Autodesk Inventor part; units mm, degrees
(part 3 of 3)
  line L1377 (0, -93.0469) -> (0, -126.0469) construction
  arc A64 (0, -126.0469) -> (6, -132.0469) centre (6, -126.0469) ccw construction
  line L1378 (16.4732, -132.0469) -> (6, -132.0469) construction
  circle A65 centre (10, -122.0469) radius 1.6 construction
  circle A66 centre (10, 47.9531) radius 1.6 construction
  circle A67 centre (27.5, -71.0469) radius 1.6 construction
  circle A68 centre (72.5, 11.9531) radius 1.6 construction
  circle A69 centre (27.5, 11.9531) radius 1.6 construction
  circle A70 centre (50, 69.0653) radius 1.6 construction
  arc A71 (58, 66.0653) -> (55, 66.0653) centre (56.5, 66.0653) ccw construction
  line L1379 (58, 66.0653) -> (58, 63.0653) construction
  arc A72 (55, 63.0653) -> (58, 63.0653) centre (56.5, 63.0653) ccw construction
  line L1380 (55, 63.0653) -> (45, 63.0653) construction
  arc A73 (42, 63.0653) -> (45, 63.0653) centre (43.5, 63.0653) ccw construction
  line L1381 (42, 63.0653) -> (42, 66.0653) construction
  arc A74 (45, 66.0653) -> (42, 66.0653) centre (43.5, 66.0653) ccw construction
  line L1382 (45, 66.0653) -> (55, 66.0653) construction
  circle A75 centre (50, 53.0653) radius 1.6 construction
  arc A76 (58, 50.0653) -> (55, 50.0653) centre (56.5, 50.0653) ccw construction
  line L1383 (58, 50.0653) -> (58, 47.0653) construction
  arc A77 (55, 47.0653) -> (58, 47.0653) centre (56.5, 47.0653) ccw construction
  line L1384 (55, 47.0653) -> (45, 47.0653) construction
  arc A78 (42, 47.0653) -> (45, 47.0653) centre (43.5, 47.0653) ccw construction
  line L1385 (42, 47.0653) -> (42, 50.0653) construction
  arc A79 (45, 50.0653) -> (42, 50.0653) centre (43.5, 50.0653) ccw construction
  line L1386 (45, 50.0653) -> (55, 50.0653) construction
  circle A80 centre (50, 24.7653) radius 5 construction
  circle A81 centre (50, -37.0469) radius 9.5 construction
  circle A82 centre (10, 22.9531) radius 1.6 construction
  circle A83 centre (10, -97.0469) radius 1.6 construction
  circle A84 centre (10, -97.0469) radius 1.6 projected
  circle A85 centre (10, 47.9531) radius 1.6 projected
  circle A86 centre (10, 22.9531) radius 1.6 projected
  circle A87 centre (10, -122.0469) radius 1.6 projected
  line L1387 (0, 57.9531) -> (117.0753, 93.7594) projected
  line L1388 (16.0565, -177.605) -> (0, -120) projected
  arc A88 (23.9528, -184.768) -> (16.0565, -177.605) centre (25.6893, -174.92) ccw projected
  arc A89 (125, 92.8569) -> (23.9528, -184.768) centre (50, -37.0469) ccw projected
  arc A90 (117.0753, 93.7594) -> (125, 92.8569) centre (120, 84.1967) ccw projected
  circle A91 centre (50, 24.7653) radius 4 projected
  circle A92 centre (72.5, 11.9531) radius 4 projected
  circle A93 centre (27.5, -71.0469) radius 4 projected
  circle A94 centre (27.5, 11.9531) radius 4 projected
  circle A95 centre (50, -37.0469) radius 4 projected
  line L1389 (41.6494, -157.691) -> (24.8878, -97.5563)
  line L1390 (15.5661, 31.3421) -> (117.1454, 62.4091)
  line L1391 (10, 22.9531) -> (153.2744, -98.1566) construction
  arc A96 (0, 22.9531) -> (2, 16.9531) centre (10, 22.9531) ccw
  arc A97 (146.8188, -105.7937) -> (148.6361, -107.0159) centre (153.2744, -98.1566) ccw
  line L1392 (153.2744, -98.1566) -> (10, -97.0469) construction
  arc A98 (2, -91.0469) -> (2, 16.9531) centre (-69.9999, -37.0469) ccw
  arc A99 (18, -103.0469) -> (18, 28.9531) centre (-69.9999, -37.0469) ccw
  line L1393 (117.0753, 93.7594) -> (0, 57.9531) projected
  line L1394 (10, -97.0469) -> (153.2744, 24.0628) construction
  arc A100 (2, -91.0469) -> (16.4556, -104.684) centre (10, -97.0469) ccw
  line L1395 (16.4556, -104.684) -> (20, -101.6879)
  arc A101 (159.73, 16.4258) -> (162.8066, 27.0857) centre (153.2744, 24.0628) ccw
  arc A102 (147.8278, 32.4494) -> (146.8188, 31.6999) centre (153.2744, 24.0628) ccw
  arc A103 (147.8278, 32.4494) -> (117.1454, 62.4091) centre (50, -37.0469) ccw
  arc A104 (154.0392, 22.7515) -> (153.2744, 24.0628) centre (50, -37.0469) ccw
  arc A105 (41.6494, -157.691) -> (148.6361, -107.0159) centre (50, -37.0469) ccw
  arc A106 (158.1017, -89.1432) -> (158.1017, 15.0494) centre (50, -37.0469) ccw
  line L1396 (24.8878, -97.5563) -> (80.9808, -50.1409)
  line L1397 (96.1463, -37.3215) -> (158.1017, 15.0494)
  line L1398 (158.1017, -89.1432) -> (96.4712, -37.0469)
  line L1399 (88.726, -30.4999) -> (85.5678, -27.8303)
  line L1400 (80.9808, -23.9529) -> (15.5661, 31.3421)
  line L1401 (146.8188, 31.6999) -> (80.9808, -23.9529)
  line L1402 (78.0566, -26.4247) -> (3.5444, -89.4098)
  line L1403 (3.5444, 15.316) -> (78.0566, -47.6691)
  line L1404 (80.9808, -50.1409) -> (146.8188, -105.7937)
  arc A107 (10.0775, -87.0472) -> (3.5444, -89.4098) centre (10, -97.0469) ccw
  arc A108 (2, -91.0469) -> (0, -97.0469) centre (10, -97.0469) ccw
  arc A109 (22.2574, -48.4638) -> (56.5973, -66.3125) centre (50, -37.0469) ccw
  arc A110 (76.5306, -51.0514) -> (72.7156, -17.451) centre (50, -37.0469) ccw
  arc A111 (69.9978, -14.6842) -> (69.3669, -14.1357) centre (50, -37.0469) ccw
  arc A112 (52.0288, -7.1156) -> (24.5, -21.2434) centre (50, -37.0469) ccw
  line L1405 (0, 57.9531) -> (0, 22.9531)
  line L1406 (0, 18.9531) -> (0, -93.0469)
  line L1407 (0, -97.0469) -> (0, -120)
  line L1408 (0, 22.9531) -> (0, -97.0469)
  point P0 (0, 0)
  point P1 (81.6372, -37.6018)
  point P2 (81.6372, -97.6018)
  point P3 (81.6372, -36.492)
  dimension "d28" = 20
  dimension "d31" = 20
  dimension "d32" = 30
  dimension "d33" = 30
  constraints: 44 end point, 39 point on circle, 29 centre point, 29 tangent, 15 point on line, 12 parallel, 3 midpoint, 1 coincident
  measures "d28" diameter of A97
  measures "d31" radial gap between concentric circles of A98 A99
  measures "d32" distance between parallel lines of L1393 L1390
  measures "d33" distance between parallel lines of L1388 L1389
extrude "押し出し7" cut sketch "スケッチ7" against normal through all contours A96 A98 A100 L1408 L1406 | L1389 L1396 L1404 A97 A105 | L1390 A103 A102 L1401 L1400 | L1398 L1397 A106
fillet "フィレット1" radius 20 11 edges at (5, -157.691, 41.6494) (5, -107.0159, 148.6361) (5, -97.5563, 24.8878) (5, -50.1409, 80.9808) (5, -37.0469, 96.4712) (5, 15.0494, 158.1017) (5, -89.1432, 158.1017) (5, -23.9529, 80.9808) (5, 31.3421, 15.5661) (5, 62.4091, 117.1454) (5, 32.4494, 147.8278)
sketch "スケッチ8" plane through (0, 0, 0) normal (-1, 0, 0) x (0, 0, 1)
  circle A0 centre (11.4108, -171.6235) radius 2.1
  line L0 (8.5165, -176.8793) -> (20.8655, -183.6796)
  arc A1 (6.3363, -168.422) -> (8.5165, -176.8793) centre (11.4108, -171.6235) ccw
  line L1 (16.0565, -177.605) -> (11.3027, -160.5502)
  arc A2 (16.0565, -177.605) -> (23.9528, -184.768) centre (25.6893, -174.92) ccw projected
  line L2 (11.3027, -160.5502) -> (6.3363, -168.422)
  line L3 (16.0565, -177.605) -> (0, -120) projected
  circle A3 centre (11.4108, -171.6235) radius 2.1 projected
  point P0 (0, 0)
  dimension "d58" = 6
  constraints: 6 end point, 3 point on circle, 3 tangent, 2 centre point, 1 coincident, 1 collinear
  measures "d58" radius of A1
extrude "押し出し8" add sketch "スケッチ8" against normal blind 10
fillet "フィレット2" radius 20 3 edges at (5, -160.5502, 11.3027) (5, -120, 0) (5, 57.9531, 0)
sketch "スケッチ9" plane through (0, 0, 0) normal (-1, 0, 0) x (0, 0, 1)
  line L0 (8, -85.5469) -> (1, -85.5469) projected
  line L1 (1, -85.5469) -> (1, -78.5469) projected
  line L2 (1, -78.5469) -> (8, -78.5469) projected
  line L3 (8, -78.5469) -> (8, -85.5469) projected
  line L4 (9, -86.5469) -> (9, -77.5469) projected
  line L5 (9, -77.5469) -> (0, -77.5469) projected
  line L6 (0, -77.5469) -> (0, -86.5469) projected
  line L7 (0, -86.5469) -> (9, -86.5469) projected
  line L8 (184, -74.5469) -> (178, -74.5469)
  line L9 (175, -74.5469) -> (175, -77.5469)
  line L10 (178, -77.5469) -> (184, -77.5469)
  line L11 (187, -77.5469) -> (187, -74.5469)
  arc A0 (178, -74.5469) -> (175, -74.5469) centre (176.5, -74.5469) ccw
  arc A1 (175, -77.5469) -> (178, -77.5469) centre (176.5, -77.5469) ccw
  arc A2 (184, -77.5469) -> (187, -77.5469) centre (185.5, -77.5469) ccw
  arc A3 (187, -74.5469) -> (184, -74.5469) centre (185.5, -74.5469) ccw
  line L12 (8, 4.4531) -> (1, 4.4531) projected
  line L13 (1, 4.4531) -> (1, 11.4531) projected
  line L14 (1, 11.4531) -> (8, 11.4531) projected
  line L15 (8, 11.4531) -> (8, 4.4531) projected
  line L16 (9, 3.4531) -> (9, 12.4531) projected
  line L17 (9, 12.4531) -> (0, 12.4531) projected
  line L18 (0, 12.4531) -> (0, 3.4531) projected
  line L19 (0, 3.4531) -> (9, 3.4531) projected
  line L20 (184, 3.4531) -> (178, 3.4531)
  line L21 (175, 3.4531) -> (175, 0.4531)
  arc A4 (178, 3.4531) -> (175, 3.4531) centre (176.5, 3.4531) ccw
  arc A5 (175, 0.4531) -> (178, 0.4531) centre (176.5, 0.4531) ccw
  arc A6 (187, 3.4531) -> (184, 3.4531) centre (185.5, 3.4531) ccw
  line L22 (187, 0.4531) -> (187, 3.4531)
  arc A7 (184, 0.4531) -> (187, 0.4531) centre (185.5, 0.4531) ccw
  line L23 (178, 0.4531) -> (184, 0.4531)
  point P0 (0, 0)
  dimension "d41" = 3
  dimension "d42" = 12
  dimension "d43" = 166
  dimension "d44" = 3
  dimension "d45" = 3
  dimension "d46" = 3
  dimension "d47" = 3
  dimension "d52" = 78
  constraints: 16 end point, 16 point on circle, 16 point on line, 8 centre point, 2 collinear, 2 parallel, 1 horizontal, 1 perpendicular, 1 vertical, 19 other
  measures "d41" distance of L11.start L11.end
  measures "d42" distance of L9.end L11.start
  measures "d43" distance between parallel lines of L4 L9
  measures "d44" diameter of A0
  measures "d45" diameter of A1
  measures "d46" diameter of A2
  measures "d47" diameter of A3
  measures "d52" distance of L11.end L22.end
extrude "押し出し9" cut sketch "スケッチ9" against normal through all contours A3 L11 A2 L10 A1 L9 A0 L8 | A6 L22 A7 L23 A5 L21 A4 L20
